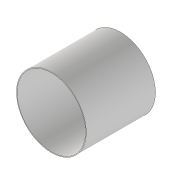
# Autodesk Inventor part: Tank_1
Saved by Autodesk Inventor 2020 (Build 240168000, 168)
## iProperties
Created: 2020-04-08
Part Number: Tank_1
Material: Generisch
Document SubType Name: Modeling
Designer: franz
Density: 1 g/cm^3
Appearance: Vorgabe
Author: franz
Autodesk Inventor part; units mm, degrees
ref_plane "YZ Plane" through (0, 0, 0) normal (1, 0, 0) x (0, 1, 0)
ref_plane "XZ Plane" through (0, 0, 0) normal (0, 1, 0) x (-1, 0, 0)
ref_plane "XY Plane" through (0, 0, 0) normal (0, 0, 1) x (1, 0, 0)
sketch "Skizze1" plane through (0, 0, 0) normal (0, 1, 0) x (-1, 0, 0)
  line L0 (0, 82.3152) -> (0, -45.1122)
  line L1 (250, 500) -> (250, 0)
  line L2 (250, 0) -> (125, 0)
  line L3 (125, 0) -> (50, -58.1376)
  line L4 (50, -58.1376) -> (50, -64.4639)
  line L5 (50, -64.4639) -> (126.711, -5)
  line L6 (126.711, -5) -> (255, -5)
  line L7 (255, -5) -> (255, 500)
  line L8 (255, 500) -> (250, 500)
  line L9 (306, 0) -> (-51, 0) projected
  point P0 (0, 0)
  dimension "d0" = 5
  dimension "d1" = 5
  dimension "d2" = 5
  dimension "d3" = 500
  dimension "d4" = 500
  dimension "d5" = 250
  dimension "d6" = 100
  constraints: 18 end point, 4 parallel, 3 vertical, 2 perpendicular, 1 collinear
  measures "d0" distance between parallel lines of L7 L1
  measures "d1" distance between parallel lines of L6 L2
  measures "d2" distance between parallel lines of L5 L3
  measures "d3" diameter of L1 L0
  measures "d4" distance of L1.start L1.end
  measures "d5" diameter of L2.end L0
  measures "d6" diameter of L4 L0
revolve "Umdrehung1" add sketch "Skizze1" angle 360 about axis through (0, 0, 82.3152) along (0, 0, -1)
sketch "Skizze2" plane through (0, 0, 0) normal (0, 0, 1) x (1, 0, 0)
  circle A0 centre (190, 0) radius 50
  circle A1 centre (0, 0) radius 250 projected
  dimension "d8" = 100
  dimension "d9" = 190
  constraints: 1 centre point
  measures "d8" diameter of A0
  measures "d9" distance of A1.centre A0.centre
extrude "Extrusion1" cut sketch "Skizze2" against normal through all contours A0
equation "\"d1\" = d0"
equation "\"d2\" = d0"
